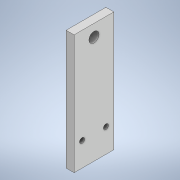
# Autodesk Inventor part: Stand
Saved by Autodesk Inventor 2022 (Build 260153000, 153)
## iProperties
Created: 2023-01-31
Part Number: Stand
Material: Generic
Document SubType Name: Modeling
Designer: Rishi  Agrawal
Density: 1 g/cm^3
Appearance: Default
Author: Rishi  Agrawal
Autodesk Inventor part; units mm, degrees
ref_plane "YZ Plane" through (0, 0, 0) normal (1, 0, 0) x (0, 1, 0)
ref_plane "XZ Plane" through (0, 0, 0) normal (0, 1, 0) x (-1, 0, 0)
ref_plane "XY Plane" through (0, 0, 0) normal (0, 0, 1) x (1, 0, 0)
sketch "Sketch2" plane through (0, 0, 0) normal (1, 0, 0) x (0, 1, 0)
  line L0 (75, 25) -> (-75, 25)
  line L1 (-75, 25) -> (-75, -25)
  line L2 (-75, -25) -> (75, -25)
  line L3 (75, -25) -> (75, 25)
  line L4 (75, 25) -> (-75, -25) construction
  line L5 (-75, 25) -> (75, -25) construction
  point P0 (0, 0)
  dimension "d4" = 150
  dimension "d5" = 50
  constraints: 12 end point, 2 midpoint, 2 parallel, 1 horizontal, 1 perpendicular
  measures "d4" distance of L2.end L1.end
  measures "d5" distance of L1.end L0.end
extrude "Extrusion" add sketch "Sketch2" along normal blind 10
sketch "Sketch3" plane through (10, 0, 0) normal (1, 0, 0) x (0, 0, -1)
  circle A0 centre (-15, -45) radius 3.2
  circle A1 centre (15, -45) radius 3.2
  circle A2 centre (0, 60) radius 6.35
  point P0 (0, 0)
  dimension "d8" = 6.4
  dimension "d9" = 12.7
  dimension "d12" = 6.4
  constraints: 3 centre point
  measures "d8" diameter of A0
  measures "d9" diameter of A2
  measures "d12" diameter of A1
extrude "Extrusion2" cut sketch "Sketch3" against normal through all
body "Solid2"
